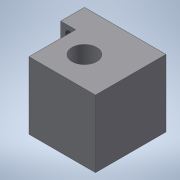
# Autodesk Inventor part: Upper Z lifter
Saved by Autodesk Inventor 2020 (Build 240168000, 168)
## iProperties
Created: 2019-05-25
Part Number: Upper Z lifter
Material: Generic
Document SubType Name: Modeling
Designer: LillaHunden
Density: 1 g/cm^3
Appearance: Default
Author: LillaHunden
Autodesk Inventor part; units mm, degrees
ref_plane "YZ Plane" through (0, 0, 0) normal (1, 0, 0) x (0, 1, 0)
ref_plane "XZ Plane" through (0, 0, 0) normal (0, 1, 0) x (-1, 0, 0)
ref_plane "XY Plane" through (0, 0, 0) normal (0, 0, 1) x (1, 0, 0)
sketch "Sketch2" plane through (0, 0, 0) normal (0, 0, 1) x (1, 0, 0)
  line L0 (-16.965, 14) -> (16.965, 14)
  line L1 (16.965, 14) -> (16.965, -14)
  line L2 (16.965, -14) -> (-16.965, -14)
  line L3 (-16.965, -14) -> (-16.965, 14)
  line L4 (-16.965, 14) -> (16.965, -14) construction
  line L5 (16.965, 14) -> (-16.965, -14) construction
  point P0 (0, 0)
  dimension "d0" = 33.93
  dimension "d1" = 28
  constraints: 12 end point, 2 midpoint, 2 parallel, 1 horizontal, 1 perpendicular
  measures "d0" distance of L1.end L2.end
  measures "d1" distance of L0.end L1.end
extrude "Extrusion1" add sketch "Sketch2" along normal blind 29.6
sketch "Sketch4" plane through (0, 0, 0) normal (0, 0, -1) x (-1, 0, 0)
  line L0 (16.965, 14) -> (16.965, -14) construction
  line L1 (-16.965, 14) -> (16.965, 14) construction
  line L2 (16.965, -14) -> (-16.965, -14) construction
  line L3 (-16.965, -14) -> (-16.965, 14) construction
  point P0 (13.485, 10.65)
  point P1 (13.665, -10.64)
  point P2 (-12.985, -10.62)
  point P3 (-13.465, 11.27)
  dimension "d11" = 3.48
  dimension "d12" = 3.3
  dimension "d13" = 3.35
  dimension "d14" = 3.36
  dimension "d15" = 3.38
  dimension "d16" = 3.98
  dimension "d17" = 3.5
  dimension "d18" = 2.73
  measures "d11" distance from line of L0 point (13.485, 10.65)
  measures "d12" distance from line of L0 point (13.665, -10.64)
  measures "d13" distance from line of L1 point (13.485, 10.65)
  measures "d14" distance from line of L2 point (13.665, -10.64)
  measures "d15" distance from line of L2 point (-12.985, -10.62)
  measures "d16" distance from line of L3 point (-12.985, -10.62)
  measures "d17" distance from line of L3 point (-13.465, 11.27)
  measures "d18" distance from line of L1 point (-13.465, 11.27)
hole "Hole1" at (13.465, 11.27, 0) at (12.985, -10.62, 0) at (-13.665, -10.64, 0) at (-13.485, 10.65, 0) direction (0, 0, 1) diameter 3.242 depth 15 tip angle 118 thread size "M4x0.7" class "6H" standard "ISO Metric profile"
sketch "Sketch3" plane through (-16.965, 14, 0) normal (0, 1, 0) x (1, 0, 0)
  circle A0 centre (16.99, -17.29) radius 5.15
  line L0 (0, 0) -> (0, -29.6) projected
  line L1 (33.93, 0) -> (0, 0) projected
  line L2 (33.93, -29.6) -> (0, -29.6) construction
  line L3 (11.84, -12.14) -> (22.14, -12.14) construction
  line L4 (22.14, -12.14) -> (22.14, -22.44) construction
  line L5 (22.14, -22.44) -> (11.84, -22.44) construction
  line L6 (11.84, -22.44) -> (11.84, -12.14) construction
  line L7 (11.84, -12.14) -> (22.14, -22.44) construction
  line L8 (22.14, -12.14) -> (11.84, -22.44) construction
  line L9 (33.93, 0) -> (33.93, -29.6) projected
  point P0 (16.965, 0)
  point P1 (0, -14.8)
  point P2 (16.965, 0)
  dimension "d4" = 10.3
  dimension "d30" = 7.16
  dimension "d32" = 11.79
  constraints: 12 end point, 4 midpoint, 2 parallel, 2 tangent, 1 centre point, 1 horizontal, 1 perpendicular
  measures "d4" diameter of A0
  measures "d30" distance between parallel lines of L2 L5
  measures "d32" distance between parallel lines of L9 L4
extrude "Extrusion2" cut sketch "Sketch3" against normal through all
sketch "Sketch5" plane through (-16.965, -14, 0) normal (-1, 0, 0) x (0, 0, 1)
  line L0 (29.6, 0) -> (29.6, 28) projected
  line L1 (22.44, 0) -> (12.14, 0) projected
  line L2 (29.6, 28) -> (10.16, 28)
  line L3 (10.16, 28) -> (10.16, 0)
  line L4 (10.16, 0) -> (29.6, 0)
  line L5 (29.6, 0) -> (29.6, 28)
  point P0 (0, 14)
  dimension "d26" = 19.44
  constraints: 8 end point, 2 parallel, 1 horizontal, 1 perpendicular, 1 point on line
  measures "d26" distance of L4.end L3.end
extrude "Extrusion3" cut sketch "Sketch5" against normal blind 6.22
move faces "Move1" translate (0, 0, 0.24) faces at (3.877, 3.4597, 0)
body "Solid1"
